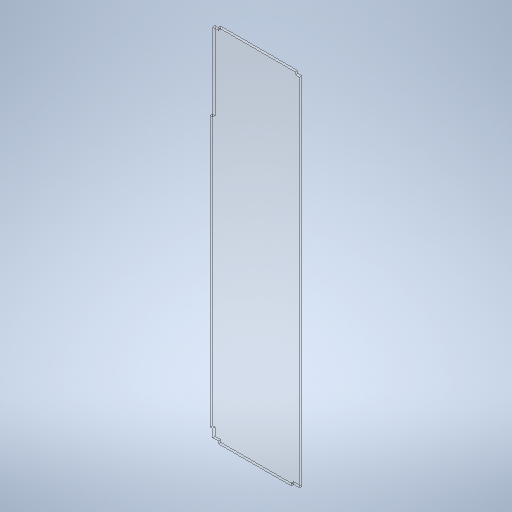
# Autodesk Inventor part: lifting cover
Saved by Autodesk Inventor 2025.4 (Build 294407000, 407)
## iProperties
Created: 2026-04-06
Part Number: lifting cover
Material: PMMA Plastic
Document SubType Name: Modeling
Designer: abdo2
Density: 1.188 g/cm^3
Appearance: Polycarbonate - Clear
Author: abdo2
Autodesk Inventor part; units mm, degrees
ref_plane "YZ Plane" through (0, 0, 0) normal (1, 0, 0) x (0, 1, 0)
ref_plane "XZ Plane" through (0, 0, 0) normal (0, 1, 0) x (-1, 0, 0)
ref_plane "XY Plane" through (0, 0, 0) normal (0, 0, 1) x (1, 0, 0)
sketch "Sketch1" plane through (0, 0, 0) normal (0, 0, 1) x (1, 0, 0)
  line L0 (0, 0) -> (0, 442)
  line L1 (0, 442) -> (110, 442)
  line L2 (110, 442) -> (110, 0)
  line L3 (110, 0) -> (0, 0)
  line L4 (10, 0) -> (10, 3)
  line L5 (10, 3) -> (0, 3)
  line L6 (100, 0) -> (100, 3)
  line L7 (100, 3) -> (110, 3)
  dimension "d0" = 442
  dimension "d1" = 110
  dimension "d4" = 3
  dimension "d5" = 90
  dimension "d6" = 10
  constraints: 16 end point, 7 perpendicular, 4 point on line, 1 vertical
  measures "d0" distance of L0.start L0.end
  measures "d1" distance of L0.end L1.end
  measures "d4" distance of L4.start L4.end
  measures "d5" distance between parallel lines of L6 L4
  measures "d6" distance between parallel lines of L0 L4
extrude "Extrusion1" add sketch "Sketch1" along normal blind 3 contours L0 L1 L2 L7 L6 L3 L4 L5
sketch "Sketch4" plane through (0, 3, 0) normal (-1, 0, 0) x (0, 0, 1)
  line L0 (3, 439) -> (3, 0) projected
  line L1 (3, 10) -> (0, 10)
  line L2 (0, 0) -> (3, 0) projected
  line L3 (0, 439) -> (0, 0) projected
  line L4 (0, 343) -> (3.087, 343)
  line L5 (0, 439) -> (3, 439) projected
  point P0 (0, -3)
  point P1 (3, 343)
  dimension "d7" = 10
  dimension "d11" = 333
  constraints: 4 end point, 2 point on line, 1 horizontal, 1 perpendicular
  measures "d7" distance between parallel lines of L2 L1
  measures "d11" distance between parallel lines of L4 L1
extrude "Extrusion2" cut sketch "Sketch4" against normal blind 3 contours L0 L2 L3 L1 | L4 L3 L5 L0
sketch "Sketch5" plane through (110, 442, 3) normal (0, 1, 0) x (1, 0, 0)
  line L0 (-10, 3) -> (0, 3) projected
  line L1 (-5, 3) -> (-5, 0)
  line L2 (-10, 0) -> (0, 0) projected
  line L3 (-100, 3) -> (-10, 3) projected
  line L4 (-100, 3) -> (-100, 0)
  line L5 (-100, 0) -> (-10, 0) projected
  line L6 (-110, 0) -> (-110, 3) projected
  dimension "d12" = 10
  constraints: 4 end point, 2 midpoint, 2 point on line, 1 vertical
  measures "d12" distance between parallel lines of L6 L4
extrude "Extrusion3" add sketch "Sketch5" along normal blind 3
body "Solid1"
